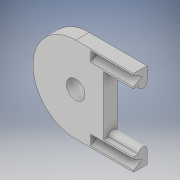
# Autodesk Inventor part: fakebattergasket1
Saved by Autodesk Inventor 2018.3 (Build 223284000, 284)
## iProperties
Created: 2019-09-05
Part Number: fakebattergasket1
Material: Generic
Document SubType Name: Modeling
Designer: Srinity
Density: 1 g/cm^3
Appearance: Default
Author: Srinity
Autodesk Inventor part; units mm, degrees
ref_plane "YZ Plane" through (0, 0, 0) normal (1, 0, 0) x (0, 1, 0)
ref_plane "XZ Plane" through (0, 0, 0) normal (0, 1, 0) x (-1, 0, 0)
ref_plane "XY Plane" through (0, 0, 0) normal (0, 0, 1) x (1, 0, 0)
sketch "Sketch1" plane through (0, 0, 0) normal (0, 0, 1) x (1, 0, 0)
  arc A0 (0, 12.7) -> (0, -12.7) centre (0, 0) ccw
  line L0 (0, 12.7) -> (17.145, 12.7)
  line L1 (17.145, 12.7) -> (17.145, -12.7)
  line L2 (17.145, -12.7) -> (0, -12.7)
  line L3 (0, -12.7) -> (0, 12.7)
  dimension "d0" = 25.4
  dimension "d7" = 17.145
  constraints: 8 end point, 2 parallel, 2 point on circle, 2 tangent, 1 centre point, 1 coincident, 1 horizontal, 1 midpoint, 1 perpendicular
  measures "d0" diameter of A0
  measures "d7" distance of L0.start L0.end
extrude "Extrusion1" add sketch "Sketch1" along normal blind 4
sketch "Sketch2" plane through (0, 0, 4) normal (0, 0, 1) x (1, 0, 0)
  circle A0 centre (0, 0) radius 2.75
  dimension "d4" = 5.5
  constraints: 1 centre point, 1 coincident
  measures "d4" diameter of A0
extrude "Extrusion2" cut sketch "Sketch2" against normal through all
sketch "Sketch3" plane through (17.145, -12.7, 0) normal (1, 0, 0) x (0, 0, -1)
  line L0 (-9.3431, 3.937) -> (-2.54, 3.937)
  line L1 (4.3638, 3.937) -> (4.3638, 21.463)
  line L2 (4.3638, 21.463) -> (0, 21.463)
  line L3 (-9.3431, 21.463) -> (-9.3431, 3.937)
  arc A0 (-2.54, 3.937) -> (0, 3.937) centre (-1.27, 3.937) ccw
  arc A1 (0, 21.463) -> (-2.54, 21.463) centre (-1.27, 21.463) ccw
  line L4 (0, 0) -> (0, 25.4) projected
  line L5 (-2.54, 3.937) -> (0, 3.937)
  line L6 (0, 3.937) -> (4.3638, 3.937)
  line L7 (0, 21.463) -> (-9.3431, 21.463)
  arc A2 (0, 3.937) -> (-2.54, 3.937) centre (-1.27, 3.937) ccw
  arc A3 (-2.54, 21.463) -> (0, 21.463) centre (-1.27, 21.463) ccw
  point P0 (0, 12.7)
  point P1 (4.3638, 12.7)
  point P2 (0, 12.7)
  dimension "d8" = 2.54
  dimension "d9" = 17.526
  constraints: 14 end point, 8 point on circle, 7 parallel, 6 point on line, 4 centre point, 3 horizontal, 3 midpoint, 3 perpendicular, 1 equal radius, 1 horizontal alignment, 1 tangent, 1 vertical alignment
  measures "d8" diameter of A0
  measures "d9" distance of L3.start L0.start
extrude "Extrusion3" cut sketch "Sketch3" against normal blind 8.89 contours L3 L7 A3 L4 A2 L0 | L4 L2 L1 L6
sketch "Sketch4" plane through (17.145, -12.7, 4) normal (1, 0, 0) x (0, 0, -1)
  line L0 (0, 0.502) -> (2.54, 1.9685)
  line L1 (2.54, 1.9685) -> (0, 3.435)
  line L2 (0, 3.435) -> (0, 21.965)
  line L3 (0, 21.965) -> (2.54, 23.4315)
  line L4 (2.54, 23.4315) -> (0, 24.898)
  line L5 (0, 24.898) -> (-1.3055, 21.2113)
  line L6 (-1.3055, 21.2113) -> (-1.3055, 1.2557)
  line L7 (-1.3055, 1.2557) -> (0, 0.502)
  line L8 (4, 0) -> (4, 3.937) projected
  line L9 (4, 21.463) -> (4, 25.4) projected
  line L10 (0, 3.937) -> (0, 21.463) projected
  point P0 (4, 12.7)
  point P1 (4, 1.9685)
  point P2 (4, 23.4315)
  point P3 (4, 23.4315)
  dimension "d12" = 60
  dimension "d13" = 60
  dimension "d14" = 120
  dimension "d15" = 120
  dimension "d16" = 2.54
  constraints: 16 end point, 3 midpoint, 3 point on line, 2 horizontal alignment, 2 vertical, 1 collinear, 1 equal length, 1 parallel
  measures "d12" angle of L1 L0
  measures "d13" angle of L4 L3
  measures "d14" angle of L1 L2
  measures "d15" angle of L3 L2
  measures "d16" distance from line of L0.end L2
extrude "Extrusion4" cut sketch "Sketch4" against normal blind 12.7
equation "\"d13\" = d12"
equation "\"d15\" = d14"
body "Solid1"
